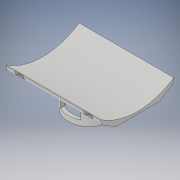
# Autodesk Inventor part: Cup_platform
Saved by Autodesk Inventor 2017 (Build 210142000, 142)
## iProperties
Created: 2018-06-16
Part Number: Cup_platform
Material: Generic
Document SubType Name: Modeling
Designer: Arthur
Density: 1 g/cm^3
Appearance: Default
Author: Arthur
Autodesk Inventor part; units mm, degrees
ref_plane "YZ Plane" through (0, 0, 0) normal (1, 0, 0) x (0, 1, 0)
ref_plane "XZ Plane" through (0, 0, 0) normal (0, 1, 0) x (-1, 0, 0)
ref_plane "XY Plane" through (0, 0, 0) normal (0, 0, 1) x (1, 0, 0)
sketch "Sketch1" plane through (0, 0, 0) normal (1, 0, 0) x (0, 1, 0)
  line L0 (-6, 25) -> (6, 25)
  line L1 (6, 25) -> (6, -25)
  line L2 (6, -25) -> (-6, -25)
  line L3 (-6, -25) -> (-6, 25)
  dimension "d0" = 12
  dimension "d1" = 50
  constraints: 8 end point, 2 parallel, 1 horizontal, 1 perpendicular
  measures "d0" distance of L1.end L2.end
  measures "d1" distance of L0.end L1.end
extrude "Extrusion1" add sketch "Sketch1" along normal blind 65
sketch "Sketch2" plane through (65, 0, 0) normal (1, 0, 0) x (0, 0, -1)
  line L0 (-25, 6) -> (-25, -6) projected
  line L1 (25, -6) -> (25, 6) projected
  line L2 (-25, 6) -> (25, 6)
  arc A0 (-25, 6) -> (25, 6) centre (0, 42.8137) ccw
  line L3 (-25, -6) -> (25, -6) projected
  line L4 (25, 3) -> (25, -6)
  line L5 (25, -6) -> (-25, -6)
  line L6 (-25, -6) -> (-25, 3)
  line L7 (0.0001, -3.2634) -> (15.0001, -3.2634)
  line L8 (15.0001, -3.2634) -> (25, 3)
  line L9 (0.0001, -3.2634) -> (-14.9999, -3.2634)
  line L10 (-14.9999, -3.2634) -> (-25, 3)
  point P0 (0, 0)
  dimension "d4" = 44.5
  dimension "d9" = 15.351
  dimension "d10" = 15.3508
  constraints: 16 end point, 3 horizontal, 2 collinear, 2 point on circle, 2 point on line, 1 centre point, 1 vertical
  measures "d4" radius of A0
  measures "d9" distance of point (0, 0) L7.end
  measures "d10" distance of point (0, 0) L9.end
extrude "Extrusion2" cut sketch "Sketch2" against normal through all contours L2 A0 | L10 L9 L7 L8 L1 L3 L0
sketch "Sketch3" plane through (65, -3.2634, -15.0001) normal (0, -1, 0) x (1, 0, 0)
  circle A0 centre (-32.5, 15) radius 15
  circle A1 centre (-32.5, 15) radius 12.5
  point P0 (-65, 15.0001)
  dimension "d14" = 25
  constraints: 2 centre point, 1 coincident
  measures "d14" diameter of A1
extrude "Extrusion3" add sketch "Sketch3" along normal blind 13
sketch "Sketch4" plane through (0, 3, 25) normal (0, 0, 1) x (1, 0, 0)
  line L0 (39.5, -15.8517) -> (25.5, -15.8517)
  line L1 (25.5, -15.8517) -> (25.5, -10.8517)
  line L2 (25.5, -10.8517) -> (39.5, -10.8517)
  line L3 (39.5, -10.8517) -> (39.5, -15.8517)
  point P0 (0, -3)
  dimension "d18" = 14
  dimension "d19" = 5
  constraints: 8 end point, 2 parallel, 1 horizontal, 1 perpendicular
  measures "d18" distance of L1.end L2.end
  measures "d19" distance of L0.end L1.end
extrude "Extrusion4" cut sketch "Sketch4" against normal through all
sketch "Sketch5" plane through (0, 3, 25) normal (0, 0, 1) x (1, 0, 0)
  line L0 (6, 0.5) -> (12, 0.5)
  line L1 (12, 0.5) -> (12, 2.5)
  line L2 (12, 2.5) -> (6, 2.5)
  line L3 (6, 2.5) -> (6, 0.5)
  line L4 (59, 0.5) -> (53, 0.5)
  line L5 (53, 0.5) -> (53, 2.5)
  line L6 (53, 2.5) -> (59, 2.5)
  line L7 (59, 2.5) -> (59, 0.5)
  point P0 (0, -3)
  point P1 (0, 0)
  point P2 (65, 0)
  dimension "d25" = 6
  dimension "d26" = 2
  dimension "d27" = 6
  dimension "d28" = 2
  constraints: 16 end point, 4 parallel, 2 horizontal, 2 perpendicular
  measures "d25" distance of L2.end L1.end
  measures "d26" distance of L1.end L0.end
  measures "d27" distance of L5.end L6.end
  measures "d28" distance of L4.end L5.end
fillet "Fillet1" radius 4 2 edges at (32.5, 3, 25) (32.5, 3, -25)
fillet "Fillet2" radius 2.5 2 edges at (32.5, -7.8517, 14.9999) (32.5, -7.8517, -15.0001)
sketch "Sketch10" plane through (65, 0, 0) normal (1, 0, 0) x (0, 0, -1)
  line L0 (-30.7469, 6.3774) -> (-5.3359, -9.5383)
  line L1 (-23.1232, 1.8245) -> (-14.9999, -3.2634) projected
  point P0 (0, 0)
  constraints: 2 end point, 1 parallel
sweep "Sweep3" cut profiles "Sketch5" path "Sketch10" path curves L0
sketch "Sketch11" plane through (65, 6, -25) normal (0, 0, -1) x (-1, 0, 0)
  line L0 (59, -0.5) -> (53, -0.5) projected
  line L1 (59, -0.5) -> (53, -0.5)
  line L2 (53, -0.5) -> (53, -2.5)
  line L3 (53, -2.5) -> (59, -2.5)
  line L4 (59, -2.5) -> (59, -0.5)
  line L5 (6, -0.5) -> (12, -0.5)
  line L6 (12, -0.5) -> (12, -2.5)
  line L7 (12, -2.5) -> (6, -2.5)
  line L8 (6, -2.5) -> (6, -0.5)
  point P0 (65, -6)
  point P1 (65, 0)
  point P2 (0, 0)
  dimension "d54" = 2
  constraints: 16 end point, 4 parallel, 2 horizontal, 2 perpendicular
  measures "d54" distance of L2.end L1.end
sketch "Sketch12" plane through (0, 0, 0) normal (-1, 0, 0) x (0, 0, 1)
  line L0 (-31.1671, 7.3521) -> (-3.1044, -10.2248)
  line L1 (-23.1233, 1.8245) -> (-15.0001, -3.2634) projected
  point P0 (0, 0)
  constraints: 2 end point, 1 parallel
sweep "Sweep4" cut profiles "Sketch11" path "Sketch12" path curves L0
body "Solid1"
